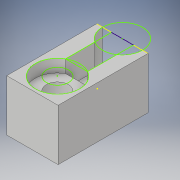
# Autodesk Inventor part: 7.2 part 2
Saved by Autodesk Inventor 2017 (Build 210142000, 142)
## iProperties
Created: 2017-03-16
Part Number: 7.2 part 2
Material: Generic
Document SubType Name: Modeling
Designer: 196918
Density: 1 g/cm^3
Appearance: Default
Author: 196918
Autodesk Inventor part; units mm, degrees
ref_plane "YZ Plane" through (0, 0, 0) normal (1, 0, 0) x (0, 1, 0)
ref_plane "XZ Plane" through (0, 0, 0) normal (0, 1, 0) x (-1, 0, 0)
ref_plane "XY Plane" through (0, 0, 0) normal (0, 0, 1) x (1, 0, 0)
sketch "Sketch1" plane through (0, 0, 0) normal (0, 1, 0) x (-1, 0, 0)
  line L0 (5.2933, 33.6678) -> (56.0933, 33.6678)
  line L1 (56.0933, 33.6678) -> (56.0933, -55.2322)
  line L2 (56.0933, -55.2322) -> (5.2933, -55.2322)
  line L3 (5.2933, -55.2322) -> (5.2933, 33.6678)
  point P0 (0, 0)
  dimension "d0" = 50.8
  dimension "d1" = 88.9
  constraints: 8 end point, 2 parallel, 1 horizontal, 1 perpendicular
  measures "d0" distance of L1.end L2.end
  measures "d1" distance of L0.end L1.end
extrude "Extrusion1" add sketch "Sketch1" along normal blind 50.8
sketch "Sketch2" plane through (0, 50.8, 0) normal (0, 1, 0) x (1, 0, 0)
  circle A0 centre (-30.6933, -8.9925) radius 21.7895
  circle A1 centre (-30.6933, -8.9925) radius 10.8785
  line L0 (-5.2933, 55.2322) -> (-56.0933, 55.2322) projected
  line L1 (-19.8148, 9.8871) -> (-41.5719, 9.8871)
  line L2 (-41.5719, 9.8871) -> (-41.5719, 55.2322)
  line L3 (-41.5719, 55.2322) -> (-19.8148, 55.2322)
  line L4 (-19.8148, 55.2322) -> (-19.8148, 9.8871)
  circle A2 centre (-30.6933, 55.2322) radius 19.7044
  point P0 (0, 0)
  constraints: 8 end point, 2 centre point, 2 parallel, 1 coincident, 1 horizontal, 1 midpoint, 1 perpendicular, 1 point on line, 3 other
extrude "Extrusion2" cut sketch "Sketch2" against normal up to next contours A2 L2 L0 L4 | L4 L0 A2 | A2 L0 L2 | L0 A2
extrude "Extrusion3" cut sketch "Sketch2" against normal blind 12.7 contours A0 L1 | L1 A0
extrude "Extrusion4" cut sketch "Sketch2" against normal blind 25.4 contours A1
extrude "Extrusion5" cut sketch "Sketch2" against normal blind 25.4 contours L1 A0 | A0 L2 A2 L4 | A2 L2 L0 L4 picked at (-29.9354, 10.8174)
body "Solid1"
